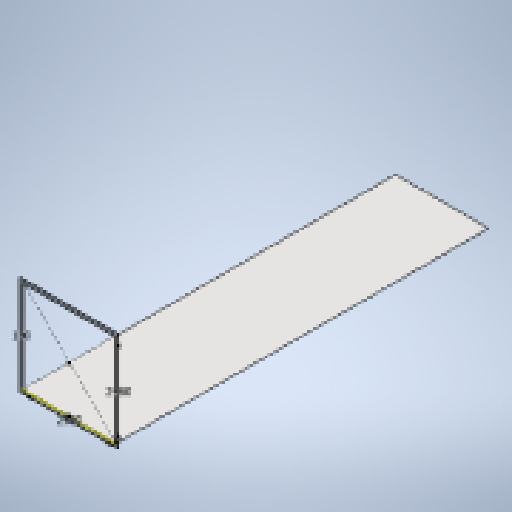
# Autodesk Inventor part: floor
Saved by Autodesk Inventor 2025.1 (Build 291241020, 241B)
## iProperties
Created: 2024-11-20
Part Number: floor
Material: Generic
Document SubType Name: Modeling
Designer: user
Density: 1 g/cm^3
Appearance: Default
Author: user
Autodesk Inventor part; units mm, degrees
ref_plane "YZ Plane" through (0, 0, 0) normal (1, 0, 0) x (0, 1, 0)
ref_plane "XZ Plane" through (0, 0, 0) normal (0, 1, 0) x (-1, 0, 0)
ref_plane "XY Plane" through (0, 0, 0) normal (0, 0, 1) x (1, 0, 0)
sketch "Sketch1" plane through (0, 0, 0) normal (0, 0, 1) x (1, 0, 0)
  line L0 (1500, -6000) -> (-1500, -6000)
  line L1 (-1500, -6000) -> (-1500, 6000)
  line L2 (-1500, 6000) -> (1500, 6000)
  line L3 (1500, 6000) -> (1500, -6000)
  line L4 (1500, -6000) -> (-1500, 6000) construction
  line L5 (-1500, -6000) -> (1500, 6000) construction
  point P0 (0, 0)
  dimension "d0" = 3000
  dimension "d1" = 12000
  constraints: 12 end point, 2 midpoint, 2 parallel, 1 horizontal, 1 perpendicular
  measures "d0" distance of L1.end L2.end
  measures "d1" distance of L0.end L1.end
extrude "Extrusion1" add sketch "Sketch1" against normal blind 10
sketch "Sketch2" plane through (-1500, -6000, 0) normal (0, -1, 0) x (1, 0, 0)
  line L0 (0, 0) -> (3000, 0) projected
  line L1 (0, 0) -> (0, -10) projected
  line L2 (3000, -10) -> (0, -10) projected
  line L3 (3000, 0) -> (3000, -10) projected
  line L4 (10, 2980) -> (2990, 2980)
  line L5 (2990, 2980) -> (2990, 0)
  line L6 (2990, 0) -> (10, 0)
  line L7 (10, 0) -> (10, 2980)
  line L8 (10, 2980) -> (2990, 0) construction
  line L9 (2990, 2980) -> (10, 0) construction
  line L10 (0, 0) -> (3000, 0) projected
  line L11 (-90, 3080) -> (3090, 3080)
  line L12 (3090, 3080) -> (3090, -100)
  line L13 (3090, -100) -> (-90, -100)
  line L14 (-90, -100) -> (-90, 3080)
  point P0 (1500, 0)
  point P1 (1500, 1490)
  point P2 (1500, 0)
  point P3 (2990, 0)
  dimension "d4" = 2980
  dimension "d5" = 2980
  dimension "d6" = 100
  constraints: 20 end point, 4 midpoint, 4 parallel, 2 perpendicular, 1 horizontal, 3 other
  measures "d4" distance of L5.end L6.end
  measures "d5" distance of L4.end L5.end
  measures "d6" distance between parallel lines of L7 L14
extrude "Extrusion2" add sketch "Sketch2" against normal blind 400
body "Solid1"
